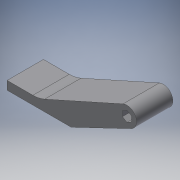
# Autodesk Inventor part: Brace
Saved by Autodesk Inventor 2019.4 (Build 234330000, 330)
## iProperties
Created: 2020-04-17
Part Number: Brace
Material: Generic
Document SubType Name: Modeling
Designer: admin
Density: 1 g/cm^3
Appearance: Default
Author: admin
Autodesk Inventor part; units mm, degrees
ref_plane "YZ Plane" through (0, 0, 0) normal (1, 0, 0) x (0, 1, 0)
ref_plane "XZ Plane" through (0, 0, 0) normal (0, 1, 0) x (-1, 0, 0)
ref_plane "XY Plane" through (0, 0, 0) normal (0, 0, 1) x (1, 0, 0)
sketch "Sketch1" plane through (0, 0, 0) normal (0, 0, 1) x (1, 0, 0)
  line L0 (92.335, -2.4537) -> (88.085, -4.9075)
  line L1 (88.085, -4.9075) -> (83.835, -2.4537)
  line L2 (83.835, -2.4537) -> (83.835, 2.4537)
  line L3 (83.835, 2.4537) -> (88.085, 4.9075)
  line L4 (88.085, 4.9075) -> (92.335, 2.4537)
  line L5 (92.335, 2.4537) -> (92.335, -2.4537)
  arc A0 (81.6015, 6.2422) -> (95.3352, -5.3324) centre (88.085, 0) ccw construction
  circle A1 centre (6.3928, -32.945) radius 22.15 projected
  arc A2 (6.3928, -59.945) -> (25.8432, -51.6715) centre (6.3928, -32.945) ccw
  line L6 (25.8432, -51.6715) -> (81.6015, 6.2422)
  line L7 (6.3928, -59.945) -> (-10.715, -59.945)
  line L8 (-10.715, -59.945) -> (-10.715, -67.945)
  line L9 (-10.715, -67.945) -> (49.285, -67.945)
  line L10 (49.285, -67.945) -> (95.3352, -5.3324)
  line L11 (-10.715, -72.945) -> (-10.715, -67.945) projected
  line L12 (58.7524, -67.945) -> (65.5572, -67.945) projected
  circle A3 centre (88.085, 0) radius 6.5 construction
  arc A4 (95.3352, -5.3324) -> (81.6015, 6.2422) centre (88.085, 0) ccw
  point P0 (0, 0)
  point P1 (92.335, 0)
  dimension "d2" = 8.5
  dimension "d13" = 18
  dimension "d16" = 8
  dimension "d17" = 60
  constraints: 22 end point, 6 point on circle, 4 tangent, 3 centre point, 2 coincident, 2 collinear, 2 perpendicular, 1 concentric, 1 horizontal, 1 midpoint, 13 other
  measures "d2" distance between parallel lines of L2 L5
  measures "d13" diameter of A0
  measures "d16" distance of L7.end L8.end
  measures "d17" distance of L8.end L9.end
extrude "Extrusion1" add sketch "Sketch1" along normal mid plane 50 contours A2 L6 A4 L10 L9 L8 L7
sketch "Sketch2" plane through (0, 0, 25) normal (0, 0, 1) x (1, 0, 0)
  line L0 (88.085, -4.9075) -> (83.835, -2.4537) projected
  line L1 (83.835, -2.4537) -> (83.835, 2.4537) projected
  line L2 (83.835, 2.4537) -> (88.085, 4.9075) projected
  line L3 (88.085, 4.9075) -> (92.335, 2.4537) projected
  line L4 (92.335, 2.4537) -> (92.335, -2.4537) projected
  line L5 (92.335, -2.4537) -> (88.085, -4.9075) projected
  line L6 (3.9734, 19.6013) -> (27.3169, 14.8693) construction
  arc A0 (88.5817, -2.4502) -> (88.5817, 2.4502) centre (88.085, 0) ccw construction
  line L7 (88.5817, -2.4502) -> (74.6189, -5.2806) construction
  arc A1 (3.9734, 19.6013) -> (3.9734, -19.6013) centre (0, 0) ccw construction
  line L8 (74.6189, 5.2806) -> (74.6189, -5.2806)
  line L9 (27.3169, 14.8693) -> (27.3169, -14.8693)
  line L10 (30.5542, 14.2131) -> (50.2765, -10.2151)
  line L11 (38.3021, 12.6425) -> (55.8449, -9.0863)
  line L12 (38.3021, 12.6425) -> (74.6189, 5.2806)
  line L13 (74.6189, 5.2806) -> (88.5817, 2.4502) construction
  line L14 (27.3169, 14.8693) -> (30.5542, 14.2131)
  line L15 (30.5542, 14.2131) -> (38.3021, 12.6425) construction
  line L16 (50.2765, -10.2151) -> (27.3169, -14.8693)
  line L17 (27.3169, -14.8693) -> (3.9734, -19.6013) construction
  line L18 (74.6189, -5.2806) -> (55.8449, -9.0863)
  line L19 (55.8449, -9.0863) -> (50.2765, -10.2151) construction
  constraints: 28 end point, 4 point on circle, 4 point on line, 2 centre point, 2 parallel, 1 vertical
extrude "Extrusion2" [suppressed]
fillet "Fillet1" [suppressed]
fillet "Fillet2" [suppressed]
sketch "Sketch3" plane through (-10.715, -59.945, 25) normal (0, 1, 0) x (1, 0, 0)
  line L0 (20, 40) -> (20, 10) construction
  circle A0 centre (20, 40) radius 2.75
  circle A1 centre (20, 10) radius 2.75
  line L1 (20, 25) -> (0, 25) construction
  line L2 (0, 0) -> (0, 50) projected
  line L3 (0, 50) -> (17.1078, 50) projected
  circle A2 centre (45, 40) radius 2.75
  circle A3 centre (45, 10) radius 2.75
  point P0 (10.715, 25)
  dimension "d18" = 5.5
  dimension "d19" = 5.5
  dimension "d20" = 30
  dimension "d21" = 20
  dimension "d24" = 25
  constraints: 4 centre point, 4 end point, 3 midpoint, 2 coincident, 2 horizontal, 1 vertical, 4 other
  measures "d18" diameter of A0
  measures "d19" diameter of A1
  measures "d20" distance of L0.start L0.end
  measures "d21" distance from line of L2 A0.centre
  measures "d24" distance of A0.centre A2.centre
extrude "Extrusion3" cut sketch "Sketch3" along normal through all both and the other way through all
sketch "Sketch4" plane through (-10.715, -59.945, 25) normal (0, 1, 0) x (1, 0, 0)
  circle A0 centre (45, 40) radius 2.75 projected
  circle A1 centre (45, 10) radius 2.75 projected
  circle A2 centre (20, 40) radius 2.75 projected
  circle A3 centre (20, 10) radius 2.75 projected
  point P0 (10.715, 25)
  constraints: 4 coincident
hole "Hole1" at (34.285, -59.945, -15) at (34.285, -59.945, 15) at (9.285, -59.945, -15) at (9.285, -59.945, 15) direction (0, 1, 0) diameter 18 end through all
fillet "Fillet3" radius 2 6 edges at (25.285, -52.2345, -15.0006) (41.6702, -35.2327, -9.8562) (29.1412, -48.2461, -22.3852) (25.285, -52.2345, 14.9994) (41.6702, -35.2327, 20.1438) (29.1412, -48.2461, 7.6148)
body "Solid1"
